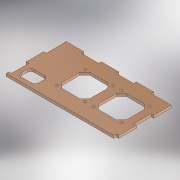
# Autodesk Inventor part: ControlBoxFace
Saved by Autodesk Inventor 2018.2 (Build 222227000, 227)
## iProperties
Created: 2018-03-30
Part Number: ControlBoxFace
Material: Wood (Birch)
Document SubType Name: Modeling
Designer: Muchen He
Density: 0.55 g/cm^3
Appearance: Birch - Natural Polished
Author: Muchen He
Autodesk Inventor part; units mm, degrees
ref_plane "YZ Plane" through (0, 0, 0) normal (1, 0, 0) x (0, 1, 0)
ref_plane "XZ Plane" through (0, 0, 0) normal (0, 1, 0) x (-1, 0, 0)
ref_plane "XY Plane" through (0, 0, 0) normal (0, 0, 1) x (1, 0, 0)
sketch "Sketch1" plane through (0, 0, 0) normal (0, 0, 1) x (1, 0, 0)
  line L0 (0, 0) -> (3, 0)
  line L1 (3, 0) -> (123, 0)
  line L2 (0, 0) -> (0, 3)
  line L3 (0, 3) -> (3, 3)
  line L4 (3, 3) -> (3, 23)
  line L5 (3, 23) -> (0, 23)
  line L6 (0, 23) -> (0, 43)
  line L7 (0, 43) -> (3, 43)
  line L8 (3, 43) -> (3, 63)
  line L9 (3, 63) -> (3, 66)
  line L10 (3, 66) -> (23, 66)
  line L11 (23, 66) -> (23, 63)
  line L12 (23, 63) -> (43, 63)
  line L13 (43, 63) -> (43, 66)
  line L14 (43, 66) -> (63, 66)
  line L15 (63, 66) -> (63, 63)
  line L16 (63, 63) -> (83, 63)
  line L17 (83, 63) -> (83, 66)
  line L18 (83, 66) -> (103, 66)
  line L19 (103, 66) -> (103, 63)
  line L20 (103, 63) -> (123, 63)
  line L21 (123, 63) -> (126, 63)
  line L22 (126, 63) -> (126, 43)
  line L23 (126, 43) -> (123, 43)
  line L24 (123, 43) -> (123, 23)
  line L25 (123, 23) -> (126, 23)
  line L26 (126, 23) -> (126, 3)
  line L27 (126, 3) -> (123, 3)
  line L28 (123, 0) -> (123, 3)
  dimension "d0" = 3
  dimension "d1" = 120
  dimension "d2" = 3
  dimension "d3" = 20
  dimension "d4" = 20
  dimension "d5" = 20
  dimension "d6" = 3
  dimension "d7" = 20
  dimension "d8" = 20
  dimension "d9" = 20
  dimension "d10" = 20
  dimension "d11" = 20
  dimension "d12" = 20
  dimension "d13" = 3
  dimension "d14" = 20
  dimension "d15" = 20
  dimension "d16" = 20
  constraints: 58 end point, 23 point on line, 12 perpendicular, 3 vertical alignment, 1 horizontal, 1 horizontal alignment, 1 vertical
  measures "d0" distance of L0.start L0.end
  measures "d1" distance of L0.end L1.end
  measures "d2" distance of L0.start L2.end
  measures "d3" distance of L3.end L4.end
  measures "d4" distance of L5.end L6.end
  measures "d5" distance of L7.end L8.end
  measures "d6" distance of L8.end L9.end
  measures "d7" distance of L9.end L10.end
  measures "d8" distance of L11.end L12.end
  measures "d9" distance of L13.end L14.end
  measures "d10" distance of L15.end L16.end
  measures "d11" distance of L17.end L18.end
  measures "d12" distance of L19.end L20.end
  measures "d13" distance of L20.end L21.end
  measures "d14" distance of L21.end L22.end
  measures "d15" distance of L23.end L24.end
  measures "d16" distance of L25.end L26.end
extrude "Extrusion1" add sketch "Sketch1" along normal blind 3
sketch "Sketch2" plane through (0, 0, 3) normal (0, 0, 1) x (1, 0, 0)
  line L0 (83, 49) -> (115, 49)
  line L1 (115, 49) -> (115, 17)
  line L2 (115, 17) -> (83, 17)
  line L3 (83, 17) -> (83, 49)
  line L4 (83, 49) -> (115, 17) construction
  line L5 (115, 49) -> (83, 17) construction
  line L6 (123, 23) -> (123, 43) construction
  circle A0 centre (83, 49) radius 1.5
  circle A1 centre (83, 17) radius 1.5
  circle A2 centre (115, 17) radius 1.5
  circle A3 centre (115, 49) radius 1.5
  line L7 (88.6569, 49) -> (83, 43.3431)
  line L8 (83, 22.6569) -> (88.6569, 17)
  line L9 (109.3431, 17) -> (115, 22.6569)
  line L10 (115, 43.3431) -> (109.3431, 49)
  point P0 (0, 0)
  point P1 (99, 33)
  point P2 (115, 33)
  point P3 (123, 33)
  dimension "d19" = 32
  dimension "d20" = 32
  dimension "d21" = 8
  dimension "d26" = 3
  dimension "d27" = 45
  dimension "d28" = 4
  constraints: 20 end point, 8 point on line, 4 centre point, 4 coincident, 4 midpoint, 4 parallel, 3 equal radius, 2 horizontal alignment, 2 perpendicular, 2 vertical alignment, 1 horizontal
  measures "d19" distance of L1.end L2.end
  measures "d20" distance of L0.end L1.end
  measures "d21" distance between parallel lines of L6 L1
  measures "d26" diameter of A3
  measures "d27" angle of L0 L10
  measures "d28" distance from line of L1.end L9
extrude "Extrusion2" cut sketch "Sketch2" against normal through all contours L3 A0 L0 | L0 A0 L3 | L0 L10 L1 L9 L2 L8 L3 L7 | A3 L1 L0 | L0 L1 A3 | A1 L2 L3 | L3 L2 A1 | A2 L2 L1 | L1 L2 A2
pattern_linear "Rectangular Pattern1" count 2 spacing 42 along (-1, 0, 0) of "Extrusion2"
sketch "Sketch3" plane through (0, 0, 3) normal (0, 0, 1) x (1, 0, 0)
  line L0 (8, 20) -> (28, 20)
  line L1 (28, 20) -> (28, 5)
  line L2 (28, 5) -> (8, 5)
  line L3 (8, 5) -> (8, 20)
  line L4 (0, 0) -> (123, 0) projected
  line L5 (3, 23) -> (3, 3) projected
  dimension "d34" = 15
  dimension "d35" = 5
  dimension "d36" = 5
  dimension "d37" = 20
  constraints: 8 end point, 2 parallel, 1 horizontal, 1 perpendicular
  measures "d34" distance of L2.end L0.start
  measures "d35" distance between parallel lines of L4 L2
  measures "d36" distance between parallel lines of L5 L3
  measures "d37" distance of L0.start L0.end
extrude "Extrusion3" cut sketch "Sketch3" against normal through all
fillet "Fillet1" radius 4 4 edges at (28, 5, 1.5) (28, 20, 1.5) (8, 20, 1.5) (8, 5, 1.5)
body "Solid1"
